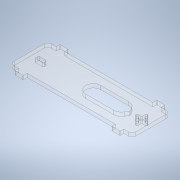
# Autodesk Inventor part: Laser-Slot-Bottom
Saved by Autodesk Inventor 2021 (Build 250183000, 183)
## iProperties
Created: 2020-06-23
Part Number: Laser-Slot-Bottom
Material: Acrylic, Clear
Document SubType Name: Modeling
Designer: lucas
Density: 1.19 g/cm^3
Appearance: Transparent - Clear
Project: 4Wire-Laser
Author: lucas
Revision Number: RLS_001
Autodesk Inventor part; units mm, degrees
ref_plane "YZ Plane" through (0, 0, 0) normal (1, 0, 0) x (0, 1, 0)
ref_plane "XZ Plane" through (0, 0, 0) normal (0, 1, 0) x (-1, 0, 0)
ref_plane "XY Plane" through (0, 0, 0) normal (0, 0, 1) x (1, 0, 0)
sketch "Sketch1" plane through (0, 0, 0) normal (0, 1, 0) x (-1, 0, 0)
  line L0 (15.892, 0.4112) -> (15.892, -0.4526)
  line L1 (15.392, -0.9526) -> (11.943, -0.9526)
  line L2 (11.943, 0.9112) -> (15.392, 0.9112)
  line L3 (15.392, 0.9112) -> (11.943, 0.9112)
  line L4 (15.892, -0.4526) -> (15.892, 0.4112)
  line L5 (15.392, -0.9526) -> (11.943, -0.9526)
  line L6 (11.943, -0.9526) -> (15.392, -0.9526)
  line L7 (-39.4963, 2.5258) -> (-39.4963, 1.1377)
  line L8 (-39.4963, -1.0763) -> (-39.4963, -2.4644)
  line L9 (-42.6438, 0.6377) -> (-41.2386, 0.6377)
  line L10 (-38.9963, 0.6377) -> (-37.5911, 0.6377)
  line L11 (-40.7386, -2.4644) -> (-40.7386, -1.0763)
  line L12 (-40.7386, 1.1377) -> (-40.7386, 2.5258)
  line L13 (-37.5911, -0.5763) -> (-38.9963, -0.5763)
  line L14 (-41.2386, -0.5763) -> (-42.6438, -0.5763)
  line L15 (-37.0911, 0.1377) -> (-37.0911, -0.0763)
  line L16 (-39.9963, -2.9644) -> (-40.2386, -2.9644)
  line L17 (-43.1438, -0.0763) -> (-43.1438, 0.1377)
  line L18 (-40.2386, 3.0258) -> (-39.9963, 3.0258)
  arc A0 (-39.4963, 2.5258) -> (-39.9963, 3.0258) centre (-39.9963, 2.5258) ccw
  arc A1 (-40.2386, 3.0258) -> (-40.7386, 2.5258) centre (-40.2386, 2.5258) ccw
  arc A2 (-41.2386, 0.6377) -> (-40.7386, 1.1377) centre (-41.2386, 1.1377) ccw
  arc A3 (-42.6438, 0.6377) -> (-43.1438, 0.1377) centre (-42.6438, 0.1377) ccw
  arc A4 (-43.1438, -0.0763) -> (-42.6438, -0.5763) centre (-42.6438, -0.0763) ccw
  arc A5 (-40.7386, -1.0763) -> (-41.2386, -0.5763) centre (-41.2386, -1.0763) ccw
  arc A6 (-40.7386, -2.4644) -> (-40.2386, -2.9644) centre (-40.2386, -2.4644) ccw
  arc A7 (-39.9963, -2.9644) -> (-39.4963, -2.4644) centre (-39.9963, -2.4644) ccw
  arc A8 (-38.9963, -0.5763) -> (-39.4963, -1.0763) centre (-38.9963, -1.0763) ccw
  arc A9 (-39.4963, 1.1377) -> (-38.9963, 0.6377) centre (-38.9963, 1.1377) ccw
  arc A10 (-37.0911, 0.1377) -> (-37.5911, 0.6377) centre (-37.5911, 0.1377) ccw
  arc A11 (-37.5911, -0.5763) -> (-37.0911, -0.0763) centre (-37.5911, -0.0763) ccw
  line L19 (-45, 8) -> (-45, -8)
  line L20 (11.443, 0.4112) -> (11.443, -0.4526)
  arc A12 (15.392, -0.9526) -> (15.892, -0.4526) centre (15.392, -0.4526) ccw
  arc A13 (15.892, 0.4112) -> (15.392, 0.9112) centre (15.392, 0.4112) ccw
  arc A14 (11.943, 0.9112) -> (11.443, 0.4112) centre (11.943, 0.4112) ccw
  arc A15 (11.443, -0.4526) -> (11.943, -0.9526) centre (11.943, -0.4526) ccw
  arc A16 (-43, 10) -> (-45, 8) centre (-43, 8) ccw
  arc A17 (-45, -8) -> (-43, -10) centre (-43, -8) ccw
  line L21 (-29.25, -2) -> (-29.25, 2) construction
  line L22 (-15, -10) -> (11, -10)
  line L23 (15.5, -10) -> (18, -10)
  line L24 (18, 10) -> (15.5, 10)
  line L25 (11, 10) -> (-30, 10)
  line L26 (-15, -10) -> (10, -10)
  line L27 (-12.5, 7) -> (-12.5, 30.9822) construction
  line L28 (-12.5, -7) -> (-12.5, -36.1495) construction
  line L29 (-30, 10) -> (-36, 10)
  line L30 (-40.5, 10) -> (-43, 10)
  line L31 (-43, -10) -> (-40.5, -10)
  line L32 (-36, -10) -> (-15, -10)
  line L33 (-43.1438, 0) -> (-43.1438, -0.0763) construction
  line L34 (-43, -10) -> (-43, -10) construction
  line L35 (20, -8) -> (20, 8)
  arc A18 (18, -10) -> (20, -8) centre (18, -8) ccw
  arc A19 (20, 8) -> (18, 10) centre (18, 8) ccw
  line L36 (15.5, -10) -> (18, -10)
  line L37 (18, 10) -> (15.5, 10)
  line L38 (15.5, -10) -> (15.5, -11.75)
  line L39 (15.25, -12) -> (11.25, -12)
  line L40 (11, -11.75) -> (11, -10)
  line L41 (15.5, 10) -> (15.5, 11.75)
  line L42 (11, 11.75) -> (11, 10)
  line L43 (-36, 10) -> (-36, 11.75)
  line L44 (-36.25, 12) -> (-40.25, 12)
  line L45 (-40.5, 11.75) -> (-40.5, 10)
  line L46 (-36, -10) -> (-36, -11.75)
  line L47 (-36.25, -12) -> (-40.25, -12)
  line L48 (-40.5, -10) -> (-40.5, -11.75)
  arc A20 (-36, 11.75) -> (-36.25, 12) centre (-36.25, 11.75) ccw
  arc A21 (-40.25, 12) -> (-40.5, 11.75) centre (-40.25, 11.75) ccw
  arc A22 (-40.5, -11.75) -> (-40.25, -12) centre (-40.25, -11.75) ccw
  arc A23 (-36.25, -12) -> (-36, -11.75) centre (-36.25, -11.75) ccw
  arc A24 (15.25, -12) -> (15.5, -11.75) centre (15.25, -11.75) ccw
  arc A25 (11, -11.75) -> (11.25, -12) centre (11.25, -11.75) ccw
  arc A26 (15.5, 11.75) -> (15.25, 12) centre (15.25, 11.75) ccw
  arc A27 (11.25, 12) -> (11, 11.75) centre (11.25, 11.75) ccw
  line L49 (11.25, 12) -> (15.25, 12)
  line L50 (-29.25, 0) -> (-14.25, 0) construction
  line L51 (-29.25, 0) -> (-14.25, 0) construction
  line L52 (-29.25, -4) -> (-14.25, -4)
  line L53 (-14.25, 4) -> (-29.25, 4)
  arc A28 (-14.25, -4) -> (-14.25, 4) centre (-14.25, 0) ccw
  line L54 (-32.6715, -2.0721) -> (-33.7507, -0.2901)
  line L55 (-33.7546, 0.2214) -> (-32.7027, 2.0197)
  arc A29 (-29.25, 4) -> (-32.7027, 2.0197) centre (-29.25, 0) ccw
  arc A30 (-32.6715, -2.0721) -> (-29.25, -4) centre (-29.25, 0) ccw
  arc A31 (-33.7546, 0.2214) -> (-33.7507, -0.2901) centre (-33.323, -0.0311) ccw
  point P0 (15.5, -12)
  point P1 (15.5, 12)
  point P2 (11, 12)
  point P3 (-36, 12)
  point P4 (-40.5, 12)
  point P5 (-36, -12)
  point P6 (-40.5, -12)
  point P7 (-21.75, 0)
  dimension "d2" = 0.5
  dimension "d4" = 0.5
  dimension "d38" = 2
  dimension "d40" = 0.25
  dimension "d41" = 47
  dimension "d42" = 47
  dimension "d43" = 56
  dimension "d44" = 15
  dimension "d45" = 15.75
  dimension "d46" = 8
  dimension "d47" = 0.5
  constraints: 114 end point, 67 tangent, 65 point on circle, 32 centre point, 23 parallel, 21 equal radius, 21 point on line, 12 perpendicular, 7 vertical, 4 horizontal, 2 midpoint, 1 collinear
  measures "d2" radius of A0
  measures "d4" radius of A12
  measures "d38" distance of L23.start point (15.5, -12)
  measures "d40" radius of A20
  measures "d41" diameter of L46 L28
  measures "d42" diameter of L43 L27
  measures "d43" distance between parallel lines of L46 L35
  measures "d44" distance of L50.start L50.end
  measures "d45" distance between parallel lines of L19 L21
  measures "d46" diameter of A28
  measures "d47" radius of A31
extrude "Extrusion1" add sketch "Sketch1" along normal blind 2
body "Solid1"
